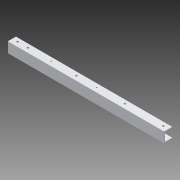
# Autodesk Inventor part: 18in C-Channel Rear
Saved by Autodesk Inventor 2013 (Build 170138000, 138)
## iProperties
Created: 2013-01-08
Part Number: 18in C-Channel Rear
Material: Aluminum 6061
Document SubType Name: Modeling
Designer: Naphat
Density: 1 g/cm^3
Author: Naphat
Autodesk Inventor part; units mm, degrees
ref_plane "YZ Plane" through (0, 0, 0) normal (1, 0, 0) x (0, 1, 0)
ref_plane "XZ Plane" through (0, 0, 0) normal (0, 1, 0) x (-1, 0, 0)
ref_plane "XY Plane" through (0, 0, 0) normal (0, 0, 1) x (1, 0, 0)
sketch "Sketch1" plane through (0, 0, 0) normal (0, 0, 1) x (1, 0, 0)
  line L0 (-16, 12.5) -> (-13, 12.5)
  line L1 (-13, 12.5) -> (-13, -9.5)
  line L2 (-13, -9.5) -> (13, -9.5)
  line L3 (13, -9.5) -> (13, 12.5)
  line L4 (13, 12.5) -> (16, 12.5)
  line L5 (16, 12.5) -> (16, -12.5)
  line L6 (16, -12.5) -> (-16, -12.5)
  line L7 (-16, -12.5) -> (-16, 12.5)
  point P0 (0, 0)
  dimension "d0" = 3
  dimension "d2" = 3
  dimension "d3" = 25
  dimension "d4" = 32
  dimension "d5" = 16
  dimension "d7" = 12.5
  dimension "d8" = 3
  dimension "d38" = 25
  constraints: 16 end point, 5 parallel, 1 collinear, 1 horizontal, 1 perpendicular
  measures "d0" distance of L0.start L0.end
  measures "d2" distance of L3.end L4.end
  measures "d3" distance of L6.end L0.start
  measures "d4" distance of L5.end L6.end
  measures "d5" distance from line of point (0, 0) L7
  measures "d7" distance from line of L6 point (0, 0)
  measures "d8" distance between parallel lines of L6 L2
  measures "d38" distance between parallel lines of L6 L4
extrude "Extrusion1" add sketch "Sketch1" against normal blind 482.6
sketch "Sketch10" plane through (16, -12.5, 0) normal (1, 0, 0) x (0, 0, -1)
  line L0 (0, 25) -> (0, 0) projected
  line L1 (482.6, 25) -> (482.6, 0) projected
  circle A0 centre (466.6, 14) radius 3.175
  circle A1 centre (16, 14) radius 3.175
  line L2 (0, 25) -> (482.6, 25) projected
  circle A2 centre (347.6, 14) radius 3.175 projected
  circle A3 centre (347.6, 14) radius 3.175
  circle A4 centre (48, 14) radius 3.175 projected
  circle A5 centre (197.8, 14) radius 3.175
  point P0 (0, 12.5)
  dimension "d65" = 6.35
  dimension "d66" = 6.35
  dimension "d67" = 16
  dimension "d68" = 16
  dimension "d77" = 11
  dimension "d78" = 299.6
  dimension "d79" = 6.35
  dimension "d80" = 149.8
  constraints: 4 centre point, 2 horizontal alignment, 1 coincident, 1 concentric
  measures "d65" diameter of A0
  measures "d66" diameter of A1
  measures "d67" distance from line of A1.centre L0
  measures "d68" distance from line of A0.centre L1
  measures "d77" distance from line of L2 A0.centre
  measures "d78" distance of A2.centre A4.centre
  measures "d79" diameter of A5
  measures "d80" distance of A4.centre A5.centre
hole "Hole2" at (16, 1.5, -466.6) at (16, 1.5, -16) at (16, 1.5, -347.6) at (16, 1.5, -48) at (16, 1.5, -197.8) direction (-1, 0, 0) diameter 6.35 end through all
sketch "Sketch11" plane through (16, -12.5, 0) normal (1, 0, 0) x (0, 0, -1)
  circle A0 centre (48, 14) radius 3.175 projected
  line L0 (0, 0) -> (482.6, 0) projected
  line L1 (0, 25) -> (482.6, 25) projected
  line L2 (50, 539.4008) -> (50, 25) projected
  circle A1 centre (407.1, 298.1) radius 12.2174 construction
  line L3 (407.1, 298.1) -> (407.1, 0) construction
  line L4 (330.9, 0) -> (893.0628, 0) construction
  line L5 (330.9, 0) -> (330.9, 539.4008) construction
  line L6 (190.45, 99.5507) -> (190.45, 71.9496) construction
  line L7 (50, 99.5507) -> (190.45, 99.5507) construction
  line L8 (190.45, 99.5507) -> (330.9, 99.5507) construction
  circle A2 centre (120.225, 14) radius 2
  circle A3 centre (260.675, 14) radius 2
  point P0 (0, 12.5)
  dimension "d83" = 76.2
  dimension "d85" = 280.9
  dimension "d86" = 4
  dimension "d87" = 14
  dimension "d95" = 70.225
  dimension "d96" = 70.225
  constraints: 12 end point, 4 point on line, 2 centre point, 2 horizontal alignment, 2 perpendicular, 1 collinear, 1 equal radius, 1 horizontal, 1 parallel
  measures "d83" distance between parallel lines of L3 L5
  measures "d85" distance between parallel lines of L2 L5
  measures "d86" diameter of A2
  measures "d87" distance from line of L0 A2.centre
  measures "d95" distance from line of A2.centre L2
  measures "d96" distance from line of L5 A3.centre
hole "Hole3" at (16, 1.5, -120.225) at (16, 1.5, -260.675) direction (-1, 0, 0) diameter 4 depth 3 tip angle 118
equation "\"d2\" = d0"
equation "\"d5\" = 0.5 * d4"
equation "\"d7\" = 0.5 * d3"
equation "\"d8\" = d0"
equation "\"d80\" = 0.5 * d78"
equation "\"d95\" = 0.25 * d85"
equation "\"d96\" = d95"
body "Solid1"
